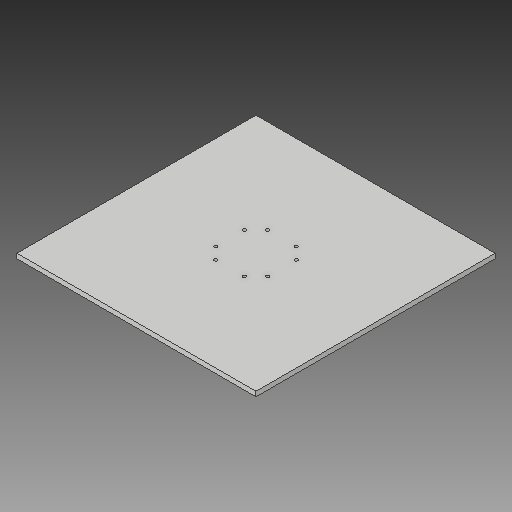
# Autodesk Inventor part: base
Saved by Autodesk Inventor 2019 (Build 230136000, 136)
## iProperties
Created: 2019-12-22
Part Number: base
Material: Типовые
Document SubType Name: Modeling
Designer: Петров Иван
Density: 1 g/cm^3
Appearance: По умолчанию
Author: Петров Иван
Autodesk Inventor part; units mm, degrees
ref_plane "YZ Plane" through (0, 0, 0) normal (1, 0, 0) x (0, 1, 0)
ref_plane "XZ Plane" through (0, 0, 0) normal (0, 1, 0) x (-1, 0, 0)
ref_plane "XY Plane" through (0, 0, 0) normal (0, 0, 1) x (1, 0, 0)
sketch "Эскиз1" plane through (0, 0, 0) normal (0, 1, 0) x (-1, 0, 0)
  line L0 (-150, 150) -> (150, 150)
  line L1 (150, 150) -> (150, -150)
  line L2 (150, -150) -> (-150, -150)
  line L3 (-150, -150) -> (-150, 150)
  line L4 (-150, 150) -> (150, -150) construction
  line L5 (150, 150) -> (-150, -150) construction
  point P0 (0, 0)
  dimension "d0" = 300
  dimension "d1" = 300
  constraints: 12 end point, 2 midpoint, 2 parallel, 1 horizontal, 1 perpendicular
  measures "d0" distance of L1.end L2.end
  measures "d1" distance of L0.end L1.end
extrude "Выдавливание1" add sketch "Эскиз1" along normal blind 6
sketch "Эскиз2" plane through (0, 6, 0) normal (0, 1, 0) x (1, 0, 0)
  circle A0 centre (-32.5, -18) radius 2
  circle A1 centre (-18, -32.5) radius 2
  line L0 (13, 27.5) -> (-13, 27.5)
  line L1 (-13, 27.5) -> (-13, 37.5)
  line L2 (-13, 37.5) -> (-23, 37.5)
  line L3 (-23, 37.5) -> (-23, 32)
  line L4 (-32, 23) -> (-23, 32)
  line L5 (-32, 23) -> (-37.5, 23)
  line L6 (-37.5, 23) -> (-37.5, 13)
  line L7 (-37.5, 13) -> (-27.5, 13)
  line L8 (-27.5, 13) -> (-27.5, -13)
  line L9 (-27.5, -13) -> (-37.5, -13)
  line L10 (-37.5, -13) -> (-37.5, -23)
  line L11 (-37.5, -23) -> (-32, -23)
  line L12 (-23, -32) -> (-32, -23)
  line L13 (-23, -32) -> (-23, -37.5)
  line L14 (-23, -37.5) -> (-13, -37.5)
  line L15 (-13, -37.5) -> (-13, -27.5)
  line L16 (-13, -27.5) -> (13, -27.5)
  line L17 (13, -27.5) -> (13, -37.5)
  line L18 (13, -37.5) -> (23, -37.5)
  line L19 (23, -37.5) -> (23, -32)
  line L20 (32, -23) -> (23, -32)
  line L21 (32, -23) -> (37.5, -23)
  line L22 (37.5, -23) -> (37.5, -13)
  line L23 (37.5, -13) -> (27.5, -13)
  line L24 (27.5, -13) -> (27.5, 13)
  line L25 (27.5, 13) -> (37.5, 13)
  line L26 (37.5, 13) -> (37.5, 23)
  line L27 (37.5, 23) -> (32, 23)
  line L28 (23, 32) -> (32, 23)
  line L29 (23, 32) -> (23, 37.5)
  line L30 (23, 37.5) -> (13, 37.5)
  line L31 (13, 37.5) -> (13, 27.5)
  circle A2 centre (-18, 32.5) radius 2
  circle A3 centre (-32.5, 18) radius 2
  circle A4 centre (18, -32.5) radius 2
  circle A5 centre (32.5, -18) radius 2
  circle A6 centre (18, 32.5) radius 2
  line L32 (-18.0075, 21.609) -> (18.0075, 21.609)
  line L33 (18.0075, 21.609) -> (21.609, 18.0075)
  line L34 (21.609, 18.0075) -> (21.609, -18.0075)
  line L35 (21.609, -18.0075) -> (18.0075, -21.609)
  line L36 (18.0075, -21.609) -> (-18.0075, -21.609)
  line L37 (-18.0075, -21.609) -> (-21.609, -18.0075)
  line L38 (-21.609, -18.0075) -> (-21.609, 18.0075)
  line L39 (-21.609, 18.0075) -> (-18.0075, 21.609)
  circle A7 centre (32.5, 18) radius 2
  arc A8 (-11.3, 0) -> (0, -11.3) centre (0, 0) ccw
  arc A9 (0, -11.3) -> (11.3, 0) centre (0, 0) ccw
  arc A10 (11.3, 0) -> (0, 11.3) centre (0, 0) ccw
  arc A11 (0, 11.3) -> (-11.3, 0) centre (0, 0) ccw
  constraints: 80 end point, 12 centre point, 8 point on circle
extrude "Выдавливание2" cut sketch "Эскиз2" against normal blind 10 contours A0 | A1 | A2 | A3 | A4 | A5 | A6 | A7
